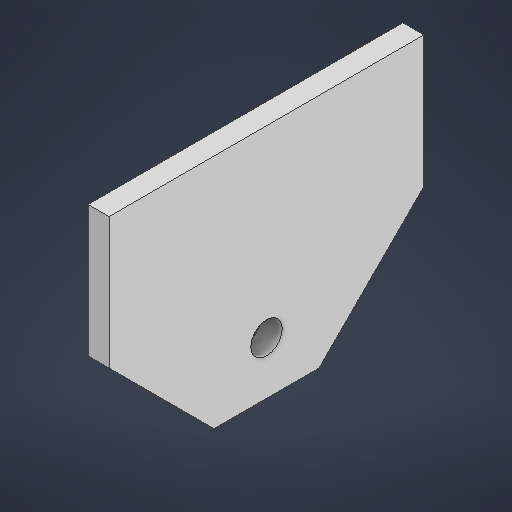
# Autodesk Inventor part: stickplate
Saved by Autodesk Inventor 2026.2 (Build 302298010, 298A)
## iProperties
Created: 2026-07-07
Part Number: stickplate
Material: Generic
Document SubType Name: Modeling
Designer: tasle
Density: 1 g/cm^3
Appearance: Default
Author: tasle
Autodesk Inventor part; units mm, degrees
ref_plane "YZ Plane" through (0, 0, 0) normal (1, 0, 0) x (0, 1, 0)
ref_plane "XZ Plane" through (0, 0, 0) normal (0, 1, 0) x (-1, 0, 0)
ref_plane "XY Plane" through (0, 0, 0) normal (0, 0, 1) x (1, 0, 0)
sketch "Sketch1" plane through (0, 0, 0) normal (1, 0, 0) x (0, 1, 0)
  line L0 (0, 0) -> (25, 0)
  line L1 (25, 0) -> (25, -60)
  line L2 (25, -60) -> (0, -60)
  line L3 (0, -60) -> (0, 0)
  line L4 (0, -20) -> (-20, -20)
  line L5 (-20, -20) -> (-20, -40)
  line L6 (-20, -40) -> (0, -40)
  line L7 (0, -40) -> (0, -20)
  line L8 (0, 0) -> (-20, -20)
  line L9 (-20, -40) -> (0, -60)
  line L10 (0, -30) -> (-20, -30)
  circle A0 centre (-10, -30) radius 3
  dimension "d0" = 25
  dimension "d1" = 60
  dimension "d2" = 20
  dimension "d3" = 20
  dimension "d4" = 6
  constraints: 22 end point, 4 midpoint, 4 parallel, 2 horizontal, 2 perpendicular, 1 centre point
  measures "d0" distance of L1.end L2.end
  measures "d1" distance of L0.end L1.end
  measures "d2" distance of L4.end L5.end
  measures "d3" distance of L5.end L6.end
  measures "d4" diameter of A0
extrude "Extrusion1" add sketch "Sketch1" along normal blind 4 contours L0 L1 L2 L3 | L3 L4 L8 | L3 L10 A0 L5 L4 | L3 L6 L5 L10 A0 | L9 L6 L3
body "Solid1"
